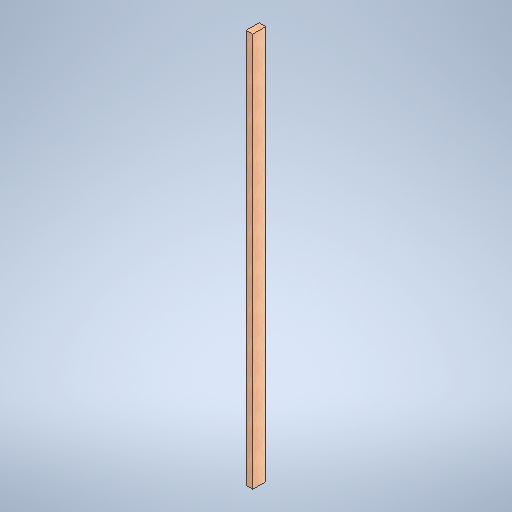
# Autodesk Inventor part: 2x4x120
Saved by Autodesk Inventor 2025 (Build 290162000, 162)
## iProperties
Created: 2024-08-29
Part Number: 2x4x120
Material: Wood (Birch)
Document SubType Name: Modeling
Designer: localadmin
Density: 0.55 g/cm^3
Appearance: Birch - Natural Medium Gloss
Author: localadmin
Autodesk Inventor part; units mm, degrees
ref_plane "YZ Plane" through (0, 0, 0) normal (1, 0, 0) x (0, 1, 0)
ref_plane "XZ Plane" through (0, 0, 0) normal (0, 1, 0) x (-1, 0, 0)
ref_plane "XY Plane" through (0, 0, 0) normal (0, 0, 1) x (1, 0, 0)
sketch "Sketch1" plane through (0, 0, 0) normal (0, 1, 0) x (-1, 0, 0)
  line L0 (25.4, 50.8) -> (-25.4, 50.8)
  line L1 (-25.4, 50.8) -> (-25.4, -50.8)
  line L2 (-25.4, -50.8) -> (25.4, -50.8)
  line L3 (25.4, -50.8) -> (25.4, 50.8)
  line L4 (25.4, 50.8) -> (-25.4, -50.8) construction
  line L5 (-25.4, 50.8) -> (25.4, -50.8) construction
  point P0 (0, 0)
  dimension "d0" = 50.8
  dimension "d1" = 101.6
  constraints: 12 end point, 2 midpoint, 2 parallel, 1 horizontal, 1 perpendicular
  measures "d0" distance of L2.end L1.end
  measures "d1" distance of L0.end L1.end
extrude "Extrusion1" add sketch "Sketch1" along normal blind 3048
body "Solid1"
